Autodesk Inventor part; units mm, degrees
(part 3 of 4)
sketch "스케치34" plane through (0, 0, 0) normal (0, -1, 0) x (1, 0, 0)
  line L0 (50.8787, 118.101) -> (84.8787, 118.101) projected
  arc A0 (87.8787, 115.101) -> (84.8787, 118.101) centre (84.8787, 115.101) ccw projected
  line L1 (87.8787, 115.101) -> (87.8787, 101.101) projected
  arc A1 (84.8787, 98.101) -> (87.8787, 101.101) centre (84.8787, 101.101) ccw projected
  line L2 (84.8787, 98.101) -> (50.8787, 98.101) projected
  arc A2 (47.8787, 101.101) -> (50.8787, 98.101) centre (50.8787, 101.101) ccw projected
  line L3 (47.8787, 101.101) -> (47.8787, 115.101) projected
  arc A3 (50.8787, 118.101) -> (47.8787, 115.101) centre (50.8787, 115.101) ccw projected
  arc A4 (-27.1, -120.9669) -> (-15.1, -132.9669) centre (-15.1, -120.9669) ccw projected
  line L4 (-15.1, -132.9669) -> (115.7787, -132.9669) projected
  arc A5 (115.7787, -132.9669) -> (127.7787, -120.9669) centre (115.7787, -120.9669) ccw projected
  line L5 (127.7787, -120.9669) -> (127.7787, -81.2883) projected
  arc A6 (127.7787, -81.2883) -> (120.2094, -70.1362) centre (115.7787, -81.2883) ccw projected
  line L6 (120.2094, -70.1362) -> (34.6692, -36.1508) projected
  arc A7 (27.1, -24.9988) -> (34.6692, -36.1508) centre (39.1, -24.9988) ccw projected
  line L7 (27.1, 24.9988) -> (27.1, -24.9988) projected
  arc A8 (34.6692, 36.1508) -> (27.1, 24.9988) centre (39.1, 24.9988) ccw projected
  line L8 (34.6692, 36.1508) -> (120.2094, 70.1362) projected
  arc A9 (120.2094, 70.1362) -> (127.7787, 81.2883) centre (115.7787, 81.2883) ccw projected
  line L9 (127.7787, 81.2883) -> (127.7787, 120.9669) projected
  arc A10 (127.7787, 120.9669) -> (115.7787, 132.9669) centre (115.7787, 120.9669) ccw projected
  line L10 (115.7787, 132.9669) -> (-15.1, 132.9669) projected
  arc A11 (-15.1, 132.9669) -> (-27.1, 120.9669) centre (-15.1, 120.9669) ccw projected
  line L11 (-27.1, 120.9669) -> (-27.1, -120.9669) projected
  circle A12 centre (99.9787, -108.101) radius 1.85 projected
  circle A13 centre (15.7787, 108.101) radius 1.85 projected
  circle A14 centre (35.7787, -108.101) radius 1.75 projected
  circle A15 centre (119.9787, 108.101) radius 1.75 projected
  circle A16 centre (119.9787, -108.101) radius 1.75 projected
  circle A17 centre (35.7787, 108.101) radius 1.75 projected
  circle A18 centre (15.7787, -108.101) radius 1.85 projected
  circle A19 centre (99.9787, 108.101) radius 1.85 projected
  circle A20 centre (0, 0) radius 8 projected
  arc A21 (13, 81.501) -> (15, 83.501) centre (13, 83.501) ccw projected
  line L12 (13, 81.501) -> (-13, 81.501) projected
  arc A22 (-15, 83.501) -> (-13, 81.501) centre (-13, 83.501) ccw projected
  line L13 (-15, 83.501) -> (-15, 93.501) projected
  arc A23 (-13, 95.501) -> (-15, 93.501) centre (-13, 93.501) ccw projected
  line L14 (-13, 95.501) -> (13, 95.501) projected
  arc A24 (15, 93.501) -> (13, 95.501) centre (13, 93.501) ccw projected
  line L15 (15, 93.501) -> (15, 83.501) projected
  circle A25 centre (49.8107, 76.501) radius 1.6 projected
  circle A26 centre (39.1, 76.501) radius 1.6 projected
  circle A27 centre (69.8107, 76.501) radius 1.6 projected
  circle A28 centre (89.8107, 76.501) radius 1.6 projected
  circle A29 centre (-4.9749, 12.0104) radius 3.1 projected
  circle A30 centre (4.9749, 12.0104) radius 3.1 projected
  circle A31 centre (-12.0104, 4.9749) radius 3.1 projected
  circle A32 centre (12.0104, 4.9749) radius 3.1 projected
  circle A33 centre (9.1, 76.501) radius 1.6 projected
  circle A34 centre (-10.9, 76.501) radius 1.6 projected
  circle A35 centre (39.1, -76.501) radius 1.6 projected
  circle A36 centre (49.8107, -76.501) radius 1.6 projected
  circle A37 centre (9.1, -76.501) radius 1.6 projected
  circle A38 centre (-10.9, -76.501) radius 1.6 projected
  circle A39 centre (69.8107, -76.501) radius 1.6 projected
  circle A40 centre (89.8107, -76.501) radius 1.6 projected
  circle A41 centre (-12.0104, -4.9749) radius 1.6 projected
  circle A42 centre (4.9749, -12.0104) radius 1.6 projected
  circle A43 centre (12.0104, -4.9749) radius 1.6 projected
  circle A44 centre (-4.9749, -12.0104) radius 1.6 projected
  line L16 (15, -83.501) -> (15, -93.501) projected
  arc A45 (13, -95.501) -> (15, -93.501) centre (13, -93.501) ccw projected
  line L17 (13, -95.501) -> (-13, -95.501) projected
  arc A46 (-15, -93.501) -> (-13, -95.501) centre (-13, -93.501) ccw projected
  line L18 (-15, -93.501) -> (-15, -83.501) projected
  arc A47 (-13, -81.501) -> (-15, -83.501) centre (-13, -83.501) ccw projected
  line L19 (-13, -81.501) -> (13, -81.501) projected
  arc A48 (15, -83.501) -> (13, -81.501) centre (13, -83.501) ccw projected
  circle A49 centre (114.8107, 76.501) radius 1.6
  line L20 (114.8107, 76.501) -> (114.8107, 78.501)
  line L21 (114.8107, 126.501) -> (114.8107, 128.501)
  line L22 (114.8107, 102.501) -> (-27.1, 102.501)
  line L23 (-27.1, 120.9669) -> (-27.1, -120.9669) projected
  circle A50 centre (89.8107, 76.501) radius 1.6 projected
  circle A51 centre (89.8107, 76.501) radius 1.6
  circle A52 centre (69.8107, 76.501) radius 1.6
  circle A53 centre (49.8107, 76.501) radius 1.6 projected
  circle A54 centre (49.8107, 76.501) radius 1.6
  circle A55 centre (39.1, 76.501) radius 1.6 projected
  circle A56 centre (39.1, 76.501) radius 1.6
  circle A57 centre (9.1, 76.501) radius 1.6 projected
  circle A58 centre (9.1, 76.501) radius 1.6
  circle A59 centre (-10.9, 76.501) radius 1.6 projected
  circle A60 centre (-10.9, 76.501) radius 1.6
  circle A61 centre (114.8107, 128.501) radius 1.6
  circle A62 centre (89.8107, 128.501) radius 1.6
  line L24 (114.8107, 128.501) -> (-24.4401, 128.501) construction
  arc A63 (-15.1, 132.9669) -> (-27.1, 120.9669) centre (-15.1, 120.9669) ccw projected
  circle A64 centre (69.8107, 128.501) radius 1.6
  circle A65 centre (49.8107, 128.501) radius 1.6
  circle A66 centre (34.8107, 128.501) radius 1.6
  circle A67 centre (4.8107, 128.501) radius 1.6
  circle A68 centre (-15.1893, 128.501) radius 1.6
  point P0 (114.8107, 127.501)
  dimension "d223" = 16.2
  dimension "d225" = 20
  dimension "d227" = 3.2
  dimension "d228" = 25
  dimension "d233" = 2
  dimension "d235" = 2
  dimension "d236" = 3.2
  dimension "d237" = 3.2
  dimension "d238" = 25
  dimension "d239" = 20
  dimension "d240" = 30
  dimension "d241" = 15
  dimension "d242" = 20
  dimension "d243" = 20
  dimension "d337" = 4.4659
  constraints: 14 centre point, 8 end point, 7 coincident, 7 point on line, 6 equal radius, 1 horizontal, 1 midpoint, 1 perpendicular, 1 point on circle, 1 vertical
  measures "d223" distance from line of L11 A34.centre
  measures "d225" distance of A28.centre A27.centre
  measures "d227" diameter of A49
  measures "d228" distance of A28.centre L20.start
  measures "d233" distance of L20.start L20.end
  measures "d235" distance of L21.start L21.end
  measures "d236" diameter of A61
  measures "d237" diameter of A62
  measures "d238" horizontal distance of point (114.811, 127.501) A62.centre
  measures "d239" distance of A67.centre A68.centre
  measures "d240" distance of A66.centre A67.centre
  measures "d241" distance of A65.centre A66.centre
  measures "d242" distance of A64.centre A65.centre
  measures "d243" distance of A62.centre A64.centre
  measures "d337" distance from line of L10 A68.centre
extrude "돌출38" cut sketch "스케치34" against normal blind 5 contours A49 | A61 | A62 | A64 | A65 | A66 | A67 | A68
mirror "미러1" about plane through (0, 0, 0) normal (0, 0, 1) of "돌출36"
mirror "미러2" about plane through (0, 0, 0) normal (0, 0, 1) of "돌출35"
mirror "미러3" about plane through (0, 0, 0) normal (0, 0, 1) of "돌출38"
fillet "모깎기8" radius 3 4 edges at (87.8787, 1.5, -98.101) (87.8787, 1.5, -118.101) (47.8787, 1.5, -98.101) (47.8787, 1.5, -118.101)
sketch "스케치35" plane through (0, 0, 0) normal (0, -1, 0) x (1, 0, 0)
  circle A0 centre (69.8107, -128.501) radius 1.6 projected
  circle A1 centre (-15.1893, -128.501) radius 1.6 projected
  circle A2 centre (4.8107, -128.501) radius 1.6 projected
  circle A3 centre (89.8107, -128.501) radius 1.6 projected
  circle A4 centre (49.8107, -128.501) radius 1.6 projected
  circle A5 centre (114.8107, -76.501) radius 1.6 projected
  circle A6 centre (34.8107, -128.501) radius 1.6 projected
  circle A7 centre (114.8107, -128.501) radius 1.6 projected
  line L0 (84.8787, -118.101) -> (50.8787, -118.101) projected
  arc A8 (47.8787, -115.101) -> (50.8787, -118.101) centre (50.8787, -115.101) ccw projected
  line L1 (47.8787, -115.101) -> (47.8787, -101.101) projected
  arc A9 (50.8787, -98.101) -> (47.8787, -101.101) centre (50.8787, -101.101) ccw projected
  line L2 (50.8787, -98.101) -> (84.8787, -98.101) projected
  arc A10 (87.8787, -101.101) -> (84.8787, -98.101) centre (84.8787, -101.101) ccw projected
  line L3 (87.8787, -101.101) -> (87.8787, -115.101) projected
  arc A11 (84.8787, -118.101) -> (87.8787, -115.101) centre (84.8787, -115.101) ccw projected
  circle A12 centre (69.8107, 128.501) radius 1.6 projected
  circle A13 centre (-15.1893, 128.501) radius 1.6 projected
  circle A14 centre (4.8107, 128.501) radius 1.6 projected
  circle A15 centre (89.8107, 128.501) radius 1.6 projected
  circle A16 centre (49.8107, 128.501) radius 1.6 projected
  circle A17 centre (114.8107, 76.501) radius 1.6 projected
  circle A18 centre (34.8107, 128.501) radius 1.6 projected
  circle A19 centre (114.8107, 128.501) radius 1.6 projected
  line L4 (50.8787, 118.101) -> (84.8787, 118.101) projected
  arc A20 (87.8787, 115.101) -> (84.8787, 118.101) centre (84.8787, 115.101) ccw projected
  line L5 (87.8787, 115.101) -> (87.8787, 101.101) projected
  arc A21 (84.8787, 98.101) -> (87.8787, 101.101) centre (84.8787, 101.101) ccw projected
  line L6 (84.8787, 98.101) -> (50.8787, 98.101) projected
  arc A22 (47.8787, 101.101) -> (50.8787, 98.101) centre (50.8787, 101.101) ccw projected
  line L7 (47.8787, 101.101) -> (47.8787, 115.101) projected
  arc A23 (50.8787, 118.101) -> (47.8787, 115.101) centre (50.8787, 115.101) ccw projected
  arc A24 (-27.1, -120.9669) -> (-15.1, -132.9669) centre (-15.1, -120.9669) ccw projected
  line L8 (-15.1, -132.9669) -> (115.7787, -132.9669) projected
  arc A25 (115.7787, -132.9669) -> (127.7787, -120.9669) centre (115.7787, -120.9669) ccw projected
  line L9 (127.7787, -120.9669) -> (127.7787, -81.2883) projected
  arc A26 (127.7787, -81.2883) -> (120.2094, -70.1362) centre (115.7787, -81.2883) ccw projected
  line L10 (120.2094, -70.1362) -> (34.6692, -36.1508) projected
  arc A27 (27.1, -24.9988) -> (34.6692, -36.1508) centre (39.1, -24.9988) ccw projected
  line L11 (27.1, 24.9988) -> (27.1, -24.9988) projected
  arc A28 (34.6692, 36.1508) -> (27.1, 24.9988) centre (39.1, 24.9988) ccw projected
  line L12 (34.6692, 36.1508) -> (120.2094, 70.1362) projected
  arc A29 (120.2094, 70.1362) -> (127.7787, 81.2883) centre (115.7787, 81.2883) ccw projected
  line L13 (127.7787, 81.2883) -> (127.7787, 120.9669) projected
  arc A30 (127.7787, 120.9669) -> (115.7787, 132.9669) centre (115.7787, 120.9669) ccw projected
  line L14 (115.7787, 132.9669) -> (-15.1, 132.9669) projected
  arc A31 (-15.1, 132.9669) -> (-27.1, 120.9669) centre (-15.1, 120.9669) ccw projected
  line L15 (-27.1, 120.9669) -> (-27.1, -120.9669) projected
  circle A32 centre (99.9787, -108.101) radius 1.85 projected
  circle A33 centre (15.7787, 108.101) radius 1.85 projected
  circle A34 centre (35.7787, -108.101) radius 1.75 projected
  circle A35 centre (119.9787, 108.101) radius 1.75 projected
  circle A36 centre (119.9787, -108.101) radius 1.75 projected
  circle A37 centre (35.7787, 108.101) radius 1.75 projected
  circle A38 centre (15.7787, -108.101) radius 1.85 projected
  circle A39 centre (99.9787, 108.101) radius 1.85 projected
  circle A40 centre (0, 0) radius 8 projected
  arc A41 (13, 81.501) -> (15, 83.501) centre (13, 83.501) ccw projected
  line L16 (13, 81.501) -> (-13, 81.501) projected
  arc A42 (-15, 83.501) -> (-13, 81.501) centre (-13, 83.501) ccw projected
  line L17 (-15, 83.501) -> (-15, 93.501) projected
  arc A43 (-13, 95.501) -> (-15, 93.501) centre (-13, 93.501) ccw projected
  line L18 (-13, 95.501) -> (13, 95.501) projected
  arc A44 (15, 93.501) -> (13, 95.501) centre (13, 93.501) ccw projected
  line L19 (15, 93.501) -> (15, 83.501) projected
  circle A45 centre (49.8107, 76.501) radius 1.6 projected
  circle A46 centre (39.1, 76.501) radius 1.6 projected
  circle A47 centre (69.8107, 76.501) radius 1.6 projected
  circle A48 centre (89.8107, 76.501) radius 1.6 projected
  circle A49 centre (-4.9749, 12.0104) radius 3.1 projected
  circle A50 centre (4.9749, 12.0104) radius 3.1 projected
  circle A51 centre (-12.0104, 4.9749) radius 3.1 projected
  circle A52 centre (12.0104, 4.9749) radius 3.1 projected
  circle A53 centre (9.1, 76.501) radius 1.6 projected
  circle A54 centre (-10.9, 76.501) radius 1.6 projected
  circle A55 centre (39.1, -76.501) radius 1.6 projected
  circle A56 centre (49.8107, -76.501) radius 1.6 projected
  circle A57 centre (9.1, -76.501) radius 1.6 projected
  circle A58 centre (-10.9, -76.501) radius 1.6 projected
  circle A59 centre (69.8107, -76.501) radius 1.6 projected
  circle A60 centre (89.8107, -76.501) radius 1.6 projected
  circle A61 centre (-12.0104, -4.9749) radius 1.6 projected
  circle A62 centre (4.9749, -12.0104) radius 1.6 projected
  circle A63 centre (12.0104, -4.9749) radius 1.6 projected
  circle A64 centre (-4.9749, -12.0104) radius 1.6 projected
  line L20 (15, -83.501) -> (15, -93.501) projected
  arc A65 (13, -95.501) -> (15, -93.501) centre (13, -93.501) ccw projected
  line L21 (13, -95.501) -> (-13, -95.501) projected
  arc A66 (-15, -93.501) -> (-13, -95.501) centre (-13, -93.501) ccw projected
  line L22 (-15, -93.501) -> (-15, -83.501) projected
  arc A67 (-13, -81.501) -> (-15, -83.501) centre (-13, -83.501) ccw projected
  line L23 (-13, -81.501) -> (13, -81.501) projected
  arc A68 (15, -83.501) -> (13, -81.501) centre (13, -83.501) ccw projected
  circle A69 centre (12.0104, 4.9749) radius 1.6
  circle A70 centre (4.9749, 12.0104) radius 1.6
  circle A71 centre (-4.9749, 12.0104) radius 1.6
  circle A72 centre (-12.0104, 4.9749) radius 3.1 projected
  circle A73 centre (-12.0104, 4.9749) radius 1.6
  dimension "d245" = 3.2
  dimension "d246" = 3.2
  dimension "d247" = 3.2
  dimension "d248" = 3.2
  constraints: 4 centre point, 4 coincident
  measures "d245" diameter of A69
  measures "d246" diameter of A70
  measures "d247" diameter of A71
  measures "d248" diameter of A73
extrude "돌출39" add sketch "스케치35" against normal blind 5 contours A49 | A50 | A51 | A52
sketch "스케치36" plane through (0, 5, 0) normal (0, 1, 0) x (1, 0, 0)
  circle A0 centre (-4.9749, -12.0104) radius 1.6 projected
  circle A1 centre (4.9749, -12.0104) radius 1.6 projected
  circle A2 centre (-12.0104, -4.9749) radius 1.6 projected
  circle A3 centre (12.0104, -4.9749) radius 1.6 projected
  circle A4 centre (69.8107, 128.501) radius 1.6 projected
  circle A5 centre (-15.1893, 128.501) radius 1.6 projected
  circle A6 centre (4.8107, 128.501) radius 1.6 projected
  circle A7 centre (89.8107, 128.501) radius 1.6 projected
  circle A8 centre (49.8107, 128.501) radius 1.6 projected
  circle A9 centre (114.8107, 76.501) radius 1.6 projected
  circle A10 centre (34.8107, 128.501) radius 1.6 projected
  circle A11 centre (114.8107, 128.501) radius 1.6 projected
  circle A12 centre (77.8787, 108.101) radius 1.8 projected
  circle A13 centre (57.8787, 108.101) radius 1.8 projected
  circle A14 centre (69.8107, -128.501) radius 1.6 projected
  circle A15 centre (-15.1893, -128.501) radius 1.6 projected
  circle A16 centre (4.8107, -128.501) radius 1.6 projected
  circle A17 centre (89.8107, -128.501) radius 1.6 projected
  circle A18 centre (49.8107, -128.501) radius 1.6 projected
  circle A19 centre (114.8107, -76.501) radius 1.6 projected
  circle A20 centre (34.8107, -128.501) radius 1.6 projected
  circle A21 centre (114.8107, -128.501) radius 1.6 projected
  circle A22 centre (77.8787, -108.101) radius 1.8 projected
  circle A23 centre (57.8787, -108.101) radius 1.8 projected
  circle A24 centre (99.9787, 108.101) radius 1.85 projected
  circle A25 centre (15.7787, -108.101) radius 1.85 projected
  circle A26 centre (35.7787, 108.101) radius 1.75 projected
  circle A27 centre (119.9787, -108.101) radius 1.75 projected
  circle A28 centre (119.9787, 108.101) radius 1.75 projected
  circle A29 centre (35.7787, -108.101) radius 1.75 projected
  circle A30 centre (15.7787, 108.101) radius 1.85 projected
  circle A31 centre (99.9787, -108.101) radius 1.85 projected
  arc A32 (-15.1, 132.9669) -> (-27.1, 120.9669) centre (-15.1, 120.9669) ccw projected
  line L0 (-27.1, 120.9669) -> (-27.1, -120.9669) projected
  arc A33 (-27.1, -120.9669) -> (-15.1, -132.9669) centre (-15.1, -120.9669) ccw projected
  line L1 (-15.1, -132.9669) -> (115.7787, -132.9669) projected
  arc A34 (115.7787, -132.9669) -> (127.7787, -120.9669) centre (115.7787, -120.9669) ccw projected
  line L2 (127.7787, -120.9669) -> (127.7787, -81.2883) projected
  arc A35 (127.7787, -81.2883) -> (120.2094, -70.1362) centre (115.7787, -81.2883) ccw projected
  line L3 (120.2094, -70.1362) -> (34.6692, -36.1508) projected
  arc A36 (27.1, -24.9988) -> (34.6692, -36.1508) centre (39.1, -24.9988) ccw projected
  line L4 (27.1, -24.9988) -> (27.1, 24.9988) projected
  arc A37 (34.6692, 36.1508) -> (27.1, 24.9988) centre (39.1, 24.9988) ccw projected
  line L5 (34.6692, 36.1508) -> (120.2094, 70.1362) projected
  arc A38 (120.2094, 70.1362) -> (127.7787, 81.2883) centre (115.7787, 81.2883) ccw projected
  line L6 (127.7787, 81.2883) -> (127.7787, 120.9669) projected
  arc A39 (127.7787, 120.9669) -> (115.7787, 132.9669) centre (115.7787, 120.9669) ccw projected
  line L7 (115.7787, 132.9669) -> (-15.1, 132.9669) projected
  arc A40 (15, -83.501) -> (13, -81.501) centre (13, -83.501) ccw projected
  line L8 (15, -83.501) -> (15, -93.501) projected
  arc A41 (13, -95.501) -> (15, -93.501) centre (13, -93.501) ccw projected
  line L9 (13, -95.501) -> (-13, -95.501) projected
  arc A42 (-15, -93.501) -> (-13, -95.501) centre (-13, -93.501) ccw projected
  line L10 (-15, -93.501) -> (-15, -83.501) projected
  arc A43 (-13, -81.501) -> (-15, -83.501) centre (-13, -83.501) ccw projected
  line L11 (-13, -81.501) -> (13, -81.501) projected
  circle A44 centre (49.8107, -76.501) radius 1.6 projected
  circle A45 centre (39.1, -76.501) radius 1.6 projected
  circle A46 centre (69.8107, -76.501) radius 1.6 projected
  circle A47 centre (89.8107, -76.501) radius 1.6 projected
  circle A48 centre (9.1, -76.501) radius 1.6 projected
  circle A49 centre (-10.9, -76.501) radius 1.6 projected
  circle A50 centre (0, 0) radius 8 projected
  line L12 (15, 93.501) -> (15, 83.501) projected
  arc A51 (13, 81.501) -> (15, 83.501) centre (13, 83.501) ccw projected
  line L13 (13, 81.501) -> (-13, 81.501) projected
  arc A52 (-15, 83.501) -> (-13, 81.501) centre (-13, 83.501) ccw projected
  line L14 (-15, 83.501) -> (-15, 93.501) projected
  arc A53 (-13, 95.501) -> (-15, 93.501) centre (-13, 93.501) ccw projected
  line L15 (-13, 95.501) -> (13, 95.501) projected
  arc A54 (15, 93.501) -> (13, 95.501) centre (13, 93.501) ccw projected
  circle A55 centre (39.1, 76.501) radius 1.6 projected
  circle A56 centre (49.8107, 76.501) radius 1.6 projected
  circle A57 centre (9.1, 76.501) radius 1.6 projected
  circle A58 centre (-10.9, 76.501) radius 1.6 projected
  circle A59 centre (69.8107, 76.501) radius 1.6 projected
  circle A60 centre (89.8107, 76.501) radius 1.6 projected
  circle A61 centre (12.0104, 4.9749) radius 3.1 projected
  circle A62 centre (-4.9749, 12.0104) radius 3.1 projected
  circle A63 centre (-12.0104, 4.9749) radius 3.1 projected
  circle A64 centre (4.9749, 12.0104) radius 3.1 projected
extrude "돌출40" add sketch "스케치36" against normal blind 5 contours A19 | A44 | A45 | A46 | A47 | A48 | A49
sketch "스케치39" plane through (0, 5, 0) normal (0, 1, 0) x (1, 0, 0)
  circle A0 centre (-4.9749, -12.0104) radius 1.6 projected
  circle A1 centre (4.9749, -12.0104) radius 1.6 projected
  circle A2 centre (-12.0104, -4.9749) radius 1.6 projected
  circle A3 centre (12.0104, -4.9749) radius 1.6 projected
  circle A4 centre (69.8107, 128.501) radius 1.6 projected
  circle A5 centre (-15.1893, 128.501) radius 1.6 projected
  circle A6 centre (4.8107, 128.501) radius 1.6 projected
  circle A7 centre (89.8107, 128.501) radius 1.6 projected
  circle A8 centre (49.8107, 128.501) radius 1.6 projected
  circle A9 centre (114.8107, 76.501) radius 1.6 projected
  circle A10 centre (34.8107, 128.501) radius 1.6 projected
  circle A11 centre (114.8107, 128.501) radius 1.6 projected
  circle A12 centre (77.8787, 108.101) radius 1.8 projected
  circle A13 centre (57.8787, 108.101) radius 1.8 projected
  circle A14 centre (69.8107, -128.501) radius 1.6 projected
  circle A15 centre (-15.1893, -128.501) radius 1.6 projected
  circle A16 centre (4.8107, -128.501) radius 1.6 projected
  circle A17 centre (89.8107, -128.501) radius 1.6 projected
  circle A18 centre (49.8107, -128.501) radius 1.6 projected
  circle A19 centre (34.8107, -128.501) radius 1.6 projected
  circle A20 centre (114.8107, -128.501) radius 1.6 projected
  circle A21 centre (77.8787, -108.101) radius 1.8 projected
  circle A22 centre (57.8787, -108.101) radius 1.8 projected
  circle A23 centre (99.9787, 108.101) radius 1.85 projected
  circle A24 centre (15.7787, -108.101) radius 1.85 projected
  circle A25 centre (35.7787, 108.101) radius 1.75 projected
  circle A26 centre (119.9787, -108.101) radius 1.75 projected
  circle A27 centre (119.9787, 108.101) radius 1.75 projected
  circle A28 centre (35.7787, -108.101) radius 1.75 projected
  circle A29 centre (15.7787, 108.101) radius 1.85 projected
  circle A30 centre (99.9787, -108.101) radius 1.85 projected
  arc A31 (-15.1, 132.9669) -> (-27.1, 120.9669) centre (-15.1, 120.9669) ccw projected
  line L0 (-27.1, 120.9669) -> (-27.1, -120.9669) projected
  arc A32 (-27.1, -120.9669) -> (-15.1, -132.9669) centre (-15.1, -120.9669) ccw projected
  line L1 (-15.1, -132.9669) -> (115.7787, -132.9669) projected
  arc A33 (115.7787, -132.9669) -> (127.7787, -120.9669) centre (115.7787, -120.9669) ccw projected
  line L2 (127.7787, -120.9669) -> (127.7787, -81.2883) projected
  arc A34 (127.7787, -81.2883) -> (120.2094, -70.1362) centre (115.7787, -81.2883) ccw projected
  line L3 (120.2094, -70.1362) -> (34.6692, -36.1508) projected
  arc A35 (27.1, -24.9988) -> (34.6692, -36.1508) centre (39.1, -24.9988) ccw projected
  line L4 (27.1, -24.9988) -> (27.1, 24.9988) projected
  arc A36 (34.6692, 36.1508) -> (27.1, 24.9988) centre (39.1, 24.9988) ccw projected
  line L5 (34.6692, 36.1508) -> (120.2094, 70.1362) projected
  arc A37 (120.2094, 70.1362) -> (127.7787, 81.2883) centre (115.7787, 81.2883) ccw projected
  line L6 (127.7787, 81.2883) -> (127.7787, 120.9669) projected
  arc A38 (127.7787, 120.9669) -> (115.7787, 132.9669) centre (115.7787, 120.9669) ccw projected
  line L7 (115.7787, 132.9669) -> (-15.1, 132.9669) projected
  arc A39 (15, -83.501) -> (13, -81.501) centre (13, -83.501) ccw projected
  line L8 (15, -83.501) -> (15, -93.501) projected
  arc A40 (13, -95.501) -> (15, -93.501) centre (13, -93.501) ccw projected
  line L9 (13, -95.501) -> (-13, -95.501) projected
  arc A41 (-15, -93.501) -> (-13, -95.501) centre (-13, -93.501) ccw projected
  line L10 (-15, -93.501) -> (-15, -83.501) projected
  arc A42 (-13, -81.501) -> (-15, -83.501) centre (-13, -83.501) ccw projected
  line L11 (-13, -81.501) -> (13, -81.501) projected
  circle A43 centre (0, 0) radius 8 projected
  line L12 (15, 93.501) -> (15, 83.501) projected
  arc A44 (13, 81.501) -> (15, 83.501) centre (13, 83.501) ccw projected
  line L13 (13, 81.501) -> (-13, 81.501) projected
  arc A45 (-15, 83.501) -> (-13, 81.501) centre (-13, 83.501) ccw projected
  line L14 (-15, 83.501) -> (-15, 93.501) projected
  arc A46 (-13, 95.501) -> (-15, 93.501) centre (-13, 93.501) ccw projected
  line L15 (-13, 95.501) -> (13, 95.501) projected
  arc A47 (15, 93.501) -> (13, 95.501) centre (13, 93.501) ccw projected
  circle A48 centre (39.1, 76.501) radius 1.6 projected
  circle A49 centre (49.8107, 76.501) radius 1.6 projected
  circle A50 centre (9.1, 76.501) radius 1.6 projected
  circle A51 centre (-10.9, 76.501) radius 1.6 projected
  circle A52 centre (69.8107, 76.501) radius 1.6 projected
  circle A53 centre (89.8107, 76.501) radius 1.6 projected
  circle A54 centre (12.0104, 4.9749) radius 3.1 projected
  circle A55 centre (-4.9749, 12.0104) radius 3.1 projected
  circle A56 centre (-12.0104, 4.9749) radius 3.1 projected
  circle A57 centre (4.9749, 12.0104) radius 3.1 projected
  line L16 (-15.1893, -128.501) -> (-15.1893, -126.501)
  line L17 (-15.1893, -126.501) -> (-15.1893, -78.501)
  line L18 (-15.1893, -78.501) -> (-15.1893, -76.501)
  circle A58 centre (-15.1893, -76.501) radius 1.6
  line L19 (-15.1893, -76.501) -> (115.7787, -76.501) construction
  circle A59 centre (4.8107, -76.501) radius 1.6
  circle A60 centre (34.8107, -76.501) radius 1.6
  circle A61 centre (49.8107, -76.501) radius 1.6
  circle A62 centre (69.8107, -76.501) radius 1.6
  circle A63 centre (89.8107, -76.501) radius 1.6
  circle A64 centre (114.8107, -76.501) radius 1.6
  dimension "d292" = 2
  dimension "d293" = 48
  dimension "d294" = 2
  dimension "d295" = 3.2
  constraints: 8 end point, 8 point on line, 7 centre point, 6 equal radius, 6 vertical alignment, 1 coincident, 1 horizontal, 1 vertical
  measures "d292" distance of L16.start L16.end
  measures "d293" distance of L16.end L17.end
  measures "d294" distance of L17.end L18.end
  measures "d295" diameter of A58
extrude "돌출41" cut sketch "스케치39" against normal blind 5 contours A58 | A59 | A60 | A61 | A62 | A63 | A64
sketch "스케치40" plane through (0, 5, 0) normal (0, 1, 0) x (1, 0, 0)
  circle A0 centre (34.8107, -76.501) radius 1.6 projected
  circle A1 centre (114.8107, -76.501) radius 1.6 projected
  circle A2 centre (49.8107, -76.501) radius 1.6 projected
  circle A3 centre (4.8107, -76.501) radius 1.6 projected
  circle A4 centre (89.8107, -76.501) radius 1.6 projected
  circle A5 centre (69.8107, -76.501) radius 1.6 projected
  circle A6 centre (-15.1893, -76.501) radius 1.6 projected
  circle A7 centre (-4.9749, -12.0104) radius 1.6 projected
  circle A8 centre (4.9749, -12.0104) radius 1.6 projected
  circle A9 centre (-12.0104, -4.9749) radius 1.6 projected
  circle A10 centre (12.0104, -4.9749) radius 1.6 projected
  circle A11 centre (69.8107, 128.501) radius 1.6 projected
  circle A12 centre (-15.1893, 128.501) radius 1.6 projected
  circle A13 centre (4.8107, 128.501) radius 1.6 projected
  circle A14 centre (89.8107, 128.501) radius 1.6 projected
  circle A15 centre (49.8107, 128.501) radius 1.6 projected
  circle A16 centre (114.8107, 76.501) radius 1.6 projected
  circle A17 centre (34.8107, 128.501) radius 1.6 projected
  circle A18 centre (114.8107, 128.501) radius 1.6 projected
  circle A19 centre (77.8787, 108.101) radius 1.8 projected
  circle A20 centre (57.8787, 108.101) radius 1.8 projected
  circle A21 centre (69.8107, -128.501) radius 1.6 projected
  circle A22 centre (-15.1893, -128.501) radius 1.6 projected
  circle A23 centre (4.8107, -128.501) radius 1.6 projected
  circle A24 centre (89.8107, -128.501) radius 1.6 projected
  circle A25 centre (49.8107, -128.501) radius 1.6 projected
  circle A26 centre (34.8107, -128.501) radius 1.6 projected
  circle A27 centre (114.8107, -128.501) radius 1.6 projected
  circle A28 centre (77.8787, -108.101) radius 1.8 projected
  circle A29 centre (57.8787, -108.101) radius 1.8 projected
  circle A30 centre (99.9787, 108.101) radius 1.85 projected
  circle A31 centre (15.7787, -108.101) radius 1.85 projected
  circle A32 centre (35.7787, 108.101) radius 1.75 projected
  circle A33 centre (119.9787, -108.101) radius 1.75 projected
  circle A34 centre (119.9787, 108.101) radius 1.75 projected
  circle A35 centre (35.7787, -108.101) radius 1.75 projected
  circle A36 centre (15.7787, 108.101) radius 1.85 projected
  circle A37 centre (99.9787, -108.101) radius 1.85 projected
  arc A38 (-15.1, 132.9669) -> (-27.1, 120.9669) centre (-15.1, 120.9669) ccw projected
  line L0 (-27.1, 120.9669) -> (-27.1, -120.9669) projected
  arc A39 (-27.1, -120.9669) -> (-15.1, -132.9669) centre (-15.1, -120.9669) ccw projected
  line L1 (-15.1, -132.9669) -> (115.7787, -132.9669) projected
  arc A40 (115.7787, -132.9669) -> (127.7787, -120.9669) centre (115.7787, -120.9669) ccw projected
  line L2 (127.7787, -120.9669) -> (127.7787, -81.2883) projected
  arc A41 (127.7787, -81.2883) -> (120.2094, -70.1362) centre (115.7787, -81.2883) ccw projected
  line L3 (120.2094, -70.1362) -> (34.6692, -36.1508) projected
  arc A42 (27.1, -24.9988) -> (34.6692, -36.1508) centre (39.1, -24.9988) ccw projected
  line L4 (27.1, -24.9988) -> (27.1, 24.9988) projected
  arc A43 (34.6692, 36.1508) -> (27.1, 24.9988) centre (39.1, 24.9988) ccw projected
  line L5 (34.6692, 36.1508) -> (120.2094, 70.1362) projected
  arc A44 (120.2094, 70.1362) -> (127.7787, 81.2883) centre (115.7787, 81.2883) ccw projected
  line L6 (127.7787, 81.2883) -> (127.7787, 120.9669) projected
  arc A45 (127.7787, 120.9669) -> (115.7787, 132.9669) centre (115.7787, 120.9669) ccw projected
  line L7 (115.7787, 132.9669) -> (-15.1, 132.9669) projected
  arc A46 (15, -83.501) -> (13, -81.501) centre (13, -83.501) ccw projected
  line L8 (15, -83.501) -> (15, -93.501) projected
  arc A47 (13, -95.501) -> (15, -93.501) centre (13, -93.501) ccw projected
  line L9 (13, -95.501) -> (-13, -95.501) projected
  arc A48 (-15, -93.501) -> (-13, -95.501) centre (-13, -93.501) ccw projected
  line L10 (-15, -93.501) -> (-15, -83.501) projected
  arc A49 (-13, -81.501) -> (-15, -83.501) centre (-13, -83.501) ccw projected
  line L11 (-13, -81.501) -> (13, -81.501) projected
  circle A50 centre (0, 0) radius 8 projected
  line L12 (15, 93.501) -> (15, 83.501) projected
  arc A51 (13, 81.501) -> (15, 83.501) centre (13, 83.501) ccw projected
  line L13 (13, 81.501) -> (-13, 81.501) projected
  arc A52 (-15, 83.501) -> (-13, 81.501) centre (-13, 83.501) ccw projected
  line L14 (-15, 83.501) -> (-15, 93.501) projected
  arc A53 (-13, 95.501) -> (-15, 93.501) centre (-13, 93.501) ccw projected
  line L15 (-13, 95.501) -> (13, 95.501) projected
  arc A54 (15, 93.501) -> (13, 95.501) centre (13, 93.501) ccw projected
  circle A55 centre (39.1, 76.501) radius 1.6 projected
  circle A56 centre (49.8107, 76.501) radius 1.6 projected
  circle A57 centre (9.1, 76.501) radius 1.6 projected
  circle A58 centre (-10.9, 76.501) radius 1.6 projected
  circle A59 centre (69.8107, 76.501) radius 1.6 projected
  circle A60 centre (89.8107, 76.501) radius 1.6 projected
  circle A61 centre (12.0104, 4.9749) radius 3.1 projected
  circle A62 centre (-4.9749, 12.0104) radius 3.1 projected
  circle A63 centre (-12.0104, 4.9749) radius 3.1 projected
  circle A64 centre (4.9749, 12.0104) radius 3.1 projected
extrude "돌출42" add sketch "스케치40" against normal blind 5 contours A11 | A12 | A13 | A14 | A15 | A16 | A17 | A18 | A55 | A56 | A57 | A58 | A59 | A60
mirror "미러4" about plane through (0, 0, 0) normal (0, 0, 1) of "돌출41", "돌출38"
chamfer "모따기4" distance 1.5 angle 45 4 edges at (-13.6104, 5, 4.9749) (-6.5749, 5, 12.0104) (3.3749, 5, 12.0104) (10.4104, 5, 4.9749)
sketch "스케치41" plane through (27.1, 0, 24.9988) normal (1, 0, 0) x (0, 0, -1)
  line L0 (49.9975, 5) -> (49.9975, 0) projected
  line L1 (49.9975, 2.5) -> (-11.1521, 2.5)
  line L2 (-11.1521, 5) -> (-11.1521, 0) projected
  line L3 (0, 0) -> (0, 5) projected
  line L4 (0, 0) -> (49.9975, 0) projected
  line L5 (49.9975, 5) -> (49.9975, 0) projected
  line L6 (0, 5) -> (49.9975, 5) projected
  circle A0 centre (32.9988, 2.5) radius 1.25 projected
  circle A1 centre (42.9988, 2.5) radius 1.25 projected
  circle A2 centre (17, 2.5) radius 1.25
  circle A3 centre (7, 2.5) radius 1.25
  circle A4 centre (32.9988, 2.5) radius 1.25 projected
  point P0 (24.9988, 0)
  point P1 (0, 2.5)
  dimension "d303" = 10
  dimension "d304" = 7
  constraints: 3 midpoint, 2 centre point, 2 end point, 2 equal radius, 2 point on line
  measures "d303" distance of A3.centre A2.centre
  measures "d304" distance of point (0, 2.5) A3.centre
extrude "돌출43" cut sketch "스케치41" against normal blind 6 contours A3 L1 | L1 A3 | A2 L1 | L1 A2
sketch "스케치42" plane through (-27.1, 5, -120.9669) normal (-1, 0, 0) x (0, 0, 1)
  line L0 (0, -5) -> (0, 0) projected
  line L1 (241.9338, -5) -> (0, -5) projected
  line L2 (241.9338, 0) -> (241.9338, -5) projected
  line L3 (0, 0) -> (241.9338, 0) projected
  circle A0 centre (112.9669, -2.5) radius 1.25 projected
  circle A1 centre (102.9669, -2.5) radius 1.25 projected
  circle A2 centre (128.9669, -2.5) radius 1.25
  circle A3 centre (138.9669, -2.5) radius 1.25
  circle A4 centre (112.9669, -2.5) radius 1.25 projected
  point P0 (120.9669, -5)
  dimension "d307" = 10
  dimension "d308" = 16
  constraints: 2 centre point, 2 equal radius
  measures "d307" distance of A3.centre A2.centre
  measures "d308" distance of A0.centre A2.centre
extrude "돌출44" cut sketch "스케치42" against normal blind 6 contours A2 | A3
sketch "스케치44" plane through (0, 0, 0) normal (0, -1, 0) x (1, 0, 0)
  circle A0 centre (114.8107, -128.501) radius 1.6 projected
  circle A1 centre (34.8107, -128.501) radius 1.6 projected
  circle A2 centre (49.8107, -128.501) radius 1.6 projected
  circle A3 centre (89.8107, -128.501) radius 1.6 projected
  circle A4 centre (4.8107, -128.501) radius 1.6 projected
  circle A5 centre (-15.1893, -128.501) radius 1.6 projected
  circle A6 centre (69.8107, -128.501) radius 1.6 projected
  circle A7 centre (-15.1893, -76.501) radius 1.6 projected
  circle A8 centre (69.8107, -76.501) radius 1.6 projected
  circle A9 centre (89.8107, -76.501) radius 1.6 projected
  circle A10 centre (4.8107, -76.501) radius 1.6 projected
  circle A11 centre (49.8107, -76.501) radius 1.6 projected
  circle A12 centre (114.8107, -76.501) radius 1.6 projected
  circle A13 centre (34.8107, -76.501) radius 1.6 projected
  circle A14 centre (34.8107, 76.501) radius 1.6 projected
  circle A15 centre (114.8107, 76.501) radius 1.6 projected
  circle A16 centre (49.8107, 76.501) radius 1.6 projected
  circle A17 centre (4.8107, 76.501) radius 1.6 projected
  circle A18 centre (89.8107, 76.501) radius 1.6 projected
  circle A19 centre (69.8107, 76.501) radius 1.6 projected
  circle A20 centre (-15.1893, 76.501) radius 1.6 projected
  circle A21 centre (-4.9749, 12.0104) radius 1.6 projected
  circle A22 centre (4.9749, 12.0104) radius 1.6 projected
  circle A23 centre (-12.0104, 4.9749) radius 1.6 projected
  circle A24 centre (12.0104, 4.9749) radius 1.6 projected
  line L0 (84.8787, -118.101) -> (50.8787, -118.101) projected
  arc A25 (47.8787, -115.101) -> (50.8787, -118.101) centre (50.8787, -115.101) ccw projected
  line L1 (47.8787, -115.101) -> (47.8787, -101.101) projected
  arc A26 (50.8787, -98.101) -> (47.8787, -101.101) centre (50.8787, -101.101) ccw projected
  line L2 (50.8787, -98.101) -> (84.8787, -98.101) projected
  arc A27 (87.8787, -101.101) -> (84.8787, -98.101) centre (84.8787, -101.101) ccw projected
  line L3 (87.8787, -101.101) -> (87.8787, -115.101) projected
  arc A28 (84.8787, -118.101) -> (87.8787, -115.101) centre (84.8787, -115.101) ccw projected
  circle A29 centre (69.8107, 128.501) radius 1.6 projected
  circle A30 centre (-15.1893, 128.501) radius 1.6 projected
  circle A31 centre (4.8107, 128.501) radius 1.6 projected
  circle A32 centre (89.8107, 128.501) radius 1.6 projected
  circle A33 centre (49.8107, 128.501) radius 1.6 projected
  circle A34 centre (34.8107, 128.501) radius 1.6 projected
  circle A35 centre (114.8107, 128.501) radius 1.6 projected
  line L4 (50.8787, 118.101) -> (84.8787, 118.101) projected
  arc A36 (87.8787, 115.101) -> (84.8787, 118.101) centre (84.8787, 115.101) ccw projected
  line L5 (87.8787, 115.101) -> (87.8787, 101.101) projected
  arc A37 (84.8787, 98.101) -> (87.8787, 101.101) centre (84.8787, 101.101) ccw projected
  line L6 (84.8787, 98.101) -> (50.8787, 98.101) projected
  arc A38 (47.8787, 101.101) -> (50.8787, 98.101) centre (50.8787, 101.101) ccw projected
  line L7 (47.8787, 101.101) -> (47.8787, 115.101) projected
  arc A39 (50.8787, 118.101) -> (47.8787, 115.101) centre (50.8787, 115.101) ccw projected
  arc A40 (-27.1, -120.9669) -> (-15.1, -132.9669) centre (-15.1, -120.9669) ccw projected
  line L8 (-15.1, -132.9669) -> (115.7787, -132.9669) projected
  arc A41 (115.7787, -132.9669) -> (127.7787, -120.9669) centre (115.7787, -120.9669) ccw projected
  line L9 (127.7787, -120.9669) -> (127.7787, -81.2883) projected
  arc A42 (127.7787, -81.2883) -> (120.2094, -70.1362) centre (115.7787, -81.2883) ccw projected
  line L10 (120.2094, -70.1362) -> (34.6692, -36.1508) projected
  arc A43 (27.1, -24.9988) -> (34.6692, -36.1508) centre (39.1, -24.9988) ccw projected
  line L11 (27.1, 24.9988) -> (27.1, -24.9988) projected
  arc A44 (34.6692, 36.1508) -> (27.1, 24.9988) centre (39.1, 24.9988) ccw projected
  line L12 (34.6692, 36.1508) -> (120.2094, 70.1362) projected
  arc A45 (120.2094, 70.1362) -> (127.7787, 81.2883) centre (115.7787, 81.2883) ccw projected
  line L13 (127.7787, 81.2883) -> (127.7787, 120.9669) projected
  arc A46 (127.7787, 120.9669) -> (115.7787, 132.9669) centre (115.7787, 120.9669) ccw projected
  line L14 (115.7787, 132.9669) -> (-15.1, 132.9669) projected
  arc A47 (-15.1, 132.9669) -> (-27.1, 120.9669) centre (-15.1, 120.9669) ccw projected
  line L15 (-27.1, 120.9669) -> (-27.1, -120.9669) projected
  circle A48 centre (99.9787, -108.101) radius 1.85 projected
  circle A49 centre (15.7787, 108.101) radius 1.85 projected
  circle A50 centre (35.7787, -108.101) radius 1.75 projected
  circle A51 centre (119.9787, 108.101) radius 1.75 projected
  circle A52 centre (119.9787, -108.101) radius 1.75 projected
  circle A53 centre (35.7787, 108.101) radius 1.75 projected
  circle A54 centre (15.7787, -108.101) radius 1.85 projected
  circle A55 centre (99.9787, 108.101) radius 1.85 projected
  circle A56 centre (0, 0) radius 8 projected
  arc A57 (13, 81.501) -> (15, 83.501) centre (13, 83.501) ccw projected
  line L16 (13, 81.501) -> (-13, 81.501) projected
  arc A58 (-15, 83.501) -> (-13, 81.501) centre (-13, 83.501) ccw projected
  line L17 (-15, 83.501) -> (-15, 93.501) projected
  arc A59 (-13, 95.501) -> (-15, 93.501) centre (-13, 93.501) ccw projected
  line L18 (-13, 95.501) -> (13, 95.501) projected
  arc A60 (15, 93.501) -> (13, 95.501) centre (13, 93.501) ccw projected
  line L19 (15, 93.501) -> (15, 83.501) projected
  circle A61 centre (-12.0104, -4.9749) radius 1.6 projected
  circle A62 centre (4.9749, -12.0104) radius 1.6 projected
  circle A63 centre (12.0104, -4.9749) radius 1.6 projected
  circle A64 centre (-4.9749, -12.0104) radius 1.6 projected
  line L20 (15, -83.501) -> (15, -93.501) projected
  arc A65 (13, -95.501) -> (15, -93.501) centre (13, -93.501) ccw projected
  line L21 (13, -95.501) -> (-13, -95.501) projected
  arc A66 (-15, -93.501) -> (-13, -95.501) centre (-13, -93.501) ccw projected
  line L22 (-15, -93.501) -> (-15, -83.501) projected
  arc A67 (-13, -81.501) -> (-15, -83.501) centre (-13, -83.501) ccw projected
  line L23 (-13, -81.501) -> (13, -81.501) projected
  arc A68 (15, -83.501) -> (13, -81.501) centre (13, -83.501) ccw projected
  circle A69 centre (-15.1893, 76.501) radius 1.6 projected
  line L24 (-15.1893, 76.501) -> (-15.1893, 74.501)
  circle A70 centre (-18.1, 59.001) radius 1.6
  circle A71 centre (17.9, 59.001) radius 1.6
  dimension "d311" = 2
  dimension "d314" = 3.2
  dimension "d315" = 3.2
  dimension "d320" = 9
  dimension "d321" = 36
  dimension "d322" = 17.5
  constraints: 2 centre point, 2 end point, 1 vertical
  measures "d311" distance of L24.start L24.end
  measures "d314" diameter of A70
  measures "d315" diameter of A71
  measures "d320" distance from line of L15 A70.centre
  measures "d321" distance of A71.centre A70.centre
  measures "d322" vertical distance of A20.centre A70.centre
extrude "돌출45" cut sketch "스케치44" against normal blind 6 contours A70 | A71
sketch "스케치45" plane through (0, 0, 0) normal (0, -1, 0) x (1, 0, 0)
  circle A0 centre (-18.1, 59.001) radius 1.6 projected
  circle A1 centre (17.9, 59.001) radius 1.6 projected
  circle A2 centre (114.8107, -128.501) radius 1.6 projected
  circle A3 centre (34.8107, -128.501) radius 1.6 projected
  circle A4 centre (49.8107, -128.501) radius 1.6 projected
  circle A5 centre (89.8107, -128.501) radius 1.6 projected
  circle A6 centre (4.8107, -128.501) radius 1.6 projected
  circle A7 centre (-15.1893, -128.501) radius 1.6 projected
  circle A8 centre (69.8107, -128.501) radius 1.6 projected
  circle A9 centre (-15.1893, -76.501) radius 1.6 projected
  circle A10 centre (69.8107, -76.501) radius 1.6 projected
  circle A11 centre (89.8107, -76.501) radius 1.6 projected
  circle A12 centre (4.8107, -76.501) radius 1.6 projected
  circle A13 centre (49.8107, -76.501) radius 1.6 projected
  circle A14 centre (114.8107, -76.501) radius 1.6 projected
  circle A15 centre (34.8107, -76.501) radius 1.6 projected
  circle A16 centre (34.8107, 76.501) radius 1.6 projected
  circle A17 centre (114.8107, 76.501) radius 1.6 projected
  circle A18 centre (49.8107, 76.501) radius 1.6 projected
  circle A19 centre (4.8107, 76.501) radius 1.6 projected
  circle A20 centre (89.8107, 76.501) radius 1.6 projected
  circle A21 centre (69.8107, 76.501) radius 1.6 projected
  circle A22 centre (-15.1893, 76.501) radius 1.6 projected
  circle A23 centre (-4.9749, 12.0104) radius 1.6 projected
  circle A24 centre (4.9749, 12.0104) radius 1.6 projected
  circle A25 centre (-12.0104, 4.9749) radius 1.6 projected
  circle A26 centre (12.0104, 4.9749) radius 1.6 projected
  line L0 (84.8787, -118.101) -> (50.8787, -118.101) projected
  arc A27 (47.8787, -115.101) -> (50.8787, -118.101) centre (50.8787, -115.101) ccw projected
  line L1 (47.8787, -115.101) -> (47.8787, -101.101) projected
  arc A28 (50.8787, -98.101) -> (47.8787, -101.101) centre (50.8787, -101.101) ccw projected
  line L2 (50.8787, -98.101) -> (84.8787, -98.101) projected
  arc A29 (87.8787, -101.101) -> (84.8787, -98.101) centre (84.8787, -101.101) ccw projected
  line L3 (87.8787, -101.101) -> (87.8787, -115.101) projected
  arc A30 (84.8787, -118.101) -> (87.8787, -115.101) centre (84.8787, -115.101) ccw projected
  circle A31 centre (69.8107, 128.501) radius 1.6 projected
  circle A32 centre (-15.1893, 128.501) radius 1.6 projected
  circle A33 centre (4.8107, 128.501) radius 1.6 projected
  circle A34 centre (89.8107, 128.501) radius 1.6 projected
  circle A35 centre (49.8107, 128.501) radius 1.6 projected
  circle A36 centre (34.8107, 128.501) radius 1.6 projected
  circle A37 centre (114.8107, 128.501) radius 1.6 projected
  line L4 (50.8787, 118.101) -> (84.8787, 118.101) projected
  arc A38 (87.8787, 115.101) -> (84.8787, 118.101) centre (84.8787, 115.101) ccw projected
  line L5 (87.8787, 115.101) -> (87.8787, 101.101) projected
  arc A39 (84.8787, 98.101) -> (87.8787, 101.101) centre (84.8787, 101.101) ccw projected
  line L6 (84.8787, 98.101) -> (50.8787, 98.101) projected
  arc A40 (47.8787, 101.101) -> (50.8787, 98.101) centre (50.8787, 101.101) ccw projected
  line L7 (47.8787, 101.101) -> (47.8787, 115.101) projected
  arc A41 (50.8787, 118.101) -> (47.8787, 115.101) centre (50.8787, 115.101) ccw projected
  arc A42 (-27.1, -120.9669) -> (-15.1, -132.9669) centre (-15.1, -120.9669) ccw projected
  line L8 (-15.1, -132.9669) -> (115.7787, -132.9669) projected
  arc A43 (115.7787, -132.9669) -> (127.7787, -120.9669) centre (115.7787, -120.9669) ccw projected
  line L9 (127.7787, -120.9669) -> (127.7787, -81.2883) projected
  arc A44 (127.7787, -81.2883) -> (120.2094, -70.1362) centre (115.7787, -81.2883) ccw projected
  line L10 (120.2094, -70.1362) -> (34.6692, -36.1508) projected
  arc A45 (27.1, -24.9988) -> (34.6692, -36.1508) centre (39.1, -24.9988) ccw projected
  line L11 (27.1, 24.9988) -> (27.1, -24.9988) projected
  arc A46 (34.6692, 36.1508) -> (27.1, 24.9988) centre (39.1, 24.9988) ccw projected
  line L12 (34.6692, 36.1508) -> (120.2094, 70.1362) projected
  arc A47 (120.2094, 70.1362) -> (127.7787, 81.2883) centre (115.7787, 81.2883) ccw projected
  line L13 (127.7787, 81.2883) -> (127.7787, 120.9669) projected
  arc A48 (127.7787, 120.9669) -> (115.7787, 132.9669) centre (115.7787, 120.9669) ccw projected
  line L14 (115.7787, 132.9669) -> (-15.1, 132.9669) projected
  arc A49 (-15.1, 132.9669) -> (-27.1, 120.9669) centre (-15.1, 120.9669) ccw projected
  line L15 (-27.1, 120.9669) -> (-27.1, -120.9669) projected
  circle A50 centre (99.9787, -108.101) radius 1.85 projected
  circle A51 centre (15.7787, 108.101) radius 1.85 projected
  circle A52 centre (35.7787, -108.101) radius 1.75 projected
  circle A53 centre (119.9787, 108.101) radius 1.75 projected
  circle A54 centre (119.9787, -108.101) radius 1.75 projected
  circle A55 centre (35.7787, 108.101) radius 1.75 projected
  circle A56 centre (15.7787, -108.101) radius 1.85 projected
  circle A57 centre (99.9787, 108.101) radius 1.85 projected
  circle A58 centre (0, 0) radius 8 projected
  arc A59 (13, 81.501) -> (15, 83.501) centre (13, 83.501) ccw projected
  line L16 (13, 81.501) -> (-13, 81.501) projected
  arc A60 (-15, 83.501) -> (-13, 81.501) centre (-13, 83.501) ccw projected
  line L17 (-15, 83.501) -> (-15, 93.501) projected
  arc A61 (-13, 95.501) -> (-15, 93.501) centre (-13, 93.501) ccw projected
  line L18 (-13, 95.501) -> (13, 95.501) projected
  arc A62 (15, 93.501) -> (13, 95.501) centre (13, 93.501) ccw projected
  line L19 (15, 93.501) -> (15, 83.501) projected
  circle A63 centre (-12.0104, -4.9749) radius 1.6 projected
  circle A64 centre (4.9749, -12.0104) radius 1.6 projected
  circle A65 centre (12.0104, -4.9749) radius 1.6 projected
  circle A66 centre (-4.9749, -12.0104) radius 1.6 projected
  line L20 (15, -83.501) -> (15, -93.501) projected
  arc A67 (13, -95.501) -> (15, -93.501) centre (13, -93.501) ccw projected
  line L21 (13, -95.501) -> (-13, -95.501) projected
  arc A68 (-15, -93.501) -> (-13, -95.501) centre (-13, -93.501) ccw projected
  line L22 (-15, -93.501) -> (-15, -83.501) projected
  arc A69 (-13, -81.501) -> (-15, -83.501) centre (-13, -83.501) ccw projected
  line L23 (-13, -81.501) -> (13, -81.501) projected
  arc A70 (15, -83.501) -> (13, -81.501) centre (13, -83.501) ccw projected
  line L24 (-27.1, 0) -> (-27.1, -28.2)
  line L25 (-27.1, -120.9669) -> (-27.1, 120.9669) projected
  line L26 (-27.1, 0) -> (-27.1, 28.2)
  arc A71 (127.7787, 120.9669) -> (115.7787, 132.9669) centre (115.7787, 120.9669) ccw projected
  line L27 (127.7787, 120.9669) -> (-30.2213, 120.9669)
  line L28 (-30.2213, 120.9669) -> (-30.2213, 28.2)
  line L29 (-30.2213, 28.2) -> (-27.1, 28.2)
  line L30 (27.1, 24.9988) -> (27.1, -24.9988) projected
  line L31 (27.1, 0) -> (-27.1, 0)
  line L32 (127.7787, -120.9669) -> (-30.2213, -120.9669)
  line L33 (-30.2213, -120.9669) -> (-30.2213, -28.2)
  line L34 (-30.2213, -28.2) -> (-27.1, -28.2)
  arc A72 (-15.1, 132.9669) -> (-27.1, 120.9669) centre (-15.1, 120.9669) ccw projected
  line L35 (-15.1, 132.9669) -> (-30.2213, 132.9669)
  line L36 (-30.2213, 132.9669) -> (-30.2213, 120.9669)
  line L37 (-30.2213, -120.9669) -> (-30.2213, -132.9669)
  line L38 (115.7787, -132.9669) -> (-15.1, -132.9669) projected
  line L39 (-30.2213, -132.9669) -> (-15.1, -132.9669)
  line L40 (-27.1, 28.2) -> (27.5349, 28.2)
  arc A73 (34.6692, 36.1508) -> (27.1, 24.9988) centre (39.1, 24.9988) ccw projected
  line L41 (-27.1, -28.2) -> (27.5349, -28.2)
  arc A74 (27.1, -24.9988) -> (34.6692, -36.1508) centre (39.1, -24.9988) ccw projected
  line L42 (27.1, 24.9988) -> (27.1, -24.9988) projected
  line L43 (27.1, -24.9988) -> (27.1, -28.2)
  line L44 (27.1, 24.9988) -> (27.1, 28.2)
  line L45 (34.6692, 36.1508) -> (34.6692, -36.1508)
  point P0 (-27.1, -28.2)
  dimension "d323" = 28.2
  dimension "d324" = 28.2
  dimension "d325" = 158
  constraints: 36 end point, 7 point on line, 5 perpendicular, 3 horizontal, 2 midpoint, 2 point on circle, 2 symmetric about line, 1 parallel, 1 tangent
  measures "d323" distance of L24.start L24.end
  measures "d324" distance of L24.start L26.end
  measures "d325" distance of L13.end L27.end
extrude "돌출46" add sketch "스케치45" against normal blind 5 contours L32 L33 L34 L15 | A42 L39 L37 L32 | L29 L28 L27 L15 | A45 L11 A46 L45 | L27 L36 L35 A49
sketch "스케치47" plane through (0, 0, 0) normal (0, -1, 0) x (1, 0, 0)
  circle A0 centre (-18.1, 59.001) radius 1.6 projected
  circle A1 centre (17.9, 59.001) radius 1.6 projected
  circle A2 centre (114.8107, -128.501) radius 1.6 projected
  circle A3 centre (34.8107, -128.501) radius 1.6 projected
  circle A4 centre (49.8107, -128.501) radius 1.6 projected
  circle A5 centre (89.8107, -128.501) radius 1.6 projected
  circle A6 centre (4.8107, -128.501) radius 1.6 projected
  circle A7 centre (-15.1893, -128.501) radius 1.6 projected
  circle A8 centre (69.8107, -128.501) radius 1.6 projected
  circle A9 centre (-15.1893, -76.501) radius 1.6 projected
  circle A10 centre (69.8107, -76.501) radius 1.6 projected
  circle A11 centre (89.8107, -76.501) radius 1.6 projected
  circle A12 centre (4.8107, -76.501) radius 1.6 projected
  circle A13 centre (49.8107, -76.501) radius 1.6 projected
  circle A14 centre (114.8107, -76.501) radius 1.6 projected
  circle A15 centre (34.8107, -76.501) radius 1.6 projected
  circle A16 centre (34.8107, 76.501) radius 1.6 projected
  circle A17 centre (114.8107, 76.501) radius 1.6 projected
  circle A18 centre (49.8107, 76.501) radius 1.6 projected
  circle A19 centre (4.8107, 76.501) radius 1.6 projected
  circle A20 centre (89.8107, 76.501) radius 1.6 projected
  circle A21 centre (69.8107, 76.501) radius 1.6 projected
  circle A22 centre (-15.1893, 76.501) radius 1.6 projected
  circle A23 centre (-4.9749, 12.0104) radius 1.6 projected
  circle A24 centre (4.9749, 12.0104) radius 1.6 projected
  circle A25 centre (-12.0104, 4.9749) radius 1.6 projected
  circle A26 centre (12.0104, 4.9749) radius 1.6 projected
  line L0 (84.8787, -118.101) -> (50.8787, -118.101) projected
  arc A27 (47.8787, -115.101) -> (50.8787, -118.101) centre (50.8787, -115.101) ccw projected
  line L1 (47.8787, -115.101) -> (47.8787, -101.101) projected
  arc A28 (50.8787, -98.101) -> (47.8787, -101.101) centre (50.8787, -101.101) ccw projected
  line L2 (50.8787, -98.101) -> (84.8787, -98.101) projected
  arc A29 (87.8787, -101.101) -> (84.8787, -98.101) centre (84.8787, -101.101) ccw projected
  line L3 (87.8787, -101.101) -> (87.8787, -115.101) projected
  arc A30 (84.8787, -118.101) -> (87.8787, -115.101) centre (84.8787, -115.101) ccw projected
  circle A31 centre (69.8107, 128.501) radius 1.6 projected
  circle A32 centre (-15.1893, 128.501) radius 1.6 projected
  circle A33 centre (4.8107, 128.501) radius 1.6 projected
  circle A34 centre (89.8107, 128.501) radius 1.6 projected
  circle A35 centre (49.8107, 128.501) radius 1.6 projected
  circle A36 centre (34.8107, 128.501) radius 1.6 projected
  circle A37 centre (114.8107, 128.501) radius 1.6 projected
  line L4 (50.8787, 118.101) -> (84.8787, 118.101) projected
  arc A38 (87.8787, 115.101) -> (84.8787, 118.101) centre (84.8787, 115.101) ccw projected
  line L5 (87.8787, 115.101) -> (87.8787, 101.101) projected
  arc A39 (84.8787, 98.101) -> (87.8787, 101.101) centre (84.8787, 101.101) ccw projected
  line L6 (84.8787, 98.101) -> (50.8787, 98.101) projected
  arc A40 (47.8787, 101.101) -> (50.8787, 98.101) centre (50.8787, 101.101) ccw projected
  line L7 (47.8787, 101.101) -> (47.8787, 115.101) projected
  arc A41 (50.8787, 118.101) -> (47.8787, 115.101) centre (50.8787, 115.101) ccw projected
  line L8 (-30.2213, -132.9669) -> (115.7787, -132.9669) projected
  arc A42 (115.7787, -132.9669) -> (127.7787, -120.9669) centre (115.7787, -120.9669) ccw projected
  line L9 (127.7787, -120.9669) -> (127.7787, -81.2883) projected
  arc A43 (127.7787, -81.2883) -> (120.2094, -70.1362) centre (115.7787, -81.2883) ccw projected
  line L10 (120.2094, -70.1362) -> (34.6692, -36.1508) projected
  line L11 (34.6692, -36.1508) -> (34.6692, 36.1508) projected
  line L12 (34.6692, 36.1508) -> (120.2094, 70.1362) projected
  arc A44 (120.2094, 70.1362) -> (127.7787, 81.2883) centre (115.7787, 81.2883) ccw projected
  line L13 (127.7787, 81.2883) -> (127.7787, 120.9669) projected
  arc A45 (127.7787, 120.9669) -> (115.7787, 132.9669) centre (115.7787, 120.9669) ccw projected
  line L14 (115.7787, 132.9669) -> (-30.2213, 132.9669) projected
  line L15 (-30.2213, 132.9669) -> (-30.2213, 28.2) projected
  line L16 (-30.2213, 28.2) -> (-27.1, 28.2) projected
  line L17 (-27.1, 28.2) -> (-27.1, -28.2) projected
  line L18 (-27.1, -28.2) -> (-30.2213, -28.2) projected
  line L19 (-30.2213, -28.2) -> (-30.2213, -132.9669) projected
  circle A46 centre (99.9787, -108.101) radius 1.85 projected
  circle A47 centre (15.7787, 108.101) radius 1.85 projected
  circle A48 centre (35.7787, -108.101) radius 1.75 projected
  circle A49 centre (119.9787, 108.101) radius 1.75 projected
  circle A50 centre (119.9787, -108.101) radius 1.75 projected
  circle A51 centre (35.7787, 108.101) radius 1.75 projected
  circle A52 centre (15.7787, -108.101) radius 1.85 projected
  circle A53 centre (99.9787, 108.101) radius 1.85 projected
  circle A54 centre (0, 0) radius 8 projected
  arc A55 (13, 81.501) -> (15, 83.501) centre (13, 83.501) ccw projected
  line L20 (13, 81.501) -> (-13, 81.501) projected
  arc A56 (-15, 83.501) -> (-13, 81.501) centre (-13, 83.501) ccw projected
  line L21 (-15, 83.501) -> (-15, 93.501) projected
  arc A57 (-13, 95.501) -> (-15, 93.501) centre (-13, 93.501) ccw projected
  line L22 (-13, 95.501) -> (13, 95.501) projected
  arc A58 (15, 93.501) -> (13, 95.501) centre (13, 93.501) ccw projected
  line L23 (15, 93.501) -> (15, 83.501) projected
  circle A59 centre (-12.0104, -4.9749) radius 1.6 projected
  circle A60 centre (4.9749, -12.0104) radius 1.6 projected
  circle A61 centre (12.0104, -4.9749) radius 1.6 projected
  circle A62 centre (-4.9749, -12.0104) radius 1.6 projected
  line L24 (15, -83.501) -> (15, -93.501) projected
  arc A63 (13, -95.501) -> (15, -93.501) centre (13, -93.501) ccw projected
  line L25 (13, -95.501) -> (-13, -95.501) projected
  arc A64 (-15, -93.501) -> (-13, -95.501) centre (-13, -93.501) ccw projected
  line L26 (-15, -93.501) -> (-15, -83.501) projected
  arc A65 (-13, -81.501) -> (-15, -83.501) centre (-13, -83.501) ccw projected
  line L27 (-13, -81.501) -> (13, -81.501) projected
  arc A66 (15, -83.501) -> (13, -81.501) centre (13, -83.501) ccw projected
  line L28 (-27.1, -28.2) -> (-27.1, 28.2) projected
  line L29 (-27.1, 0) -> (-27.1, -54.2)
  line L30 (-27.1, 0) -> (27.1, 0)
  line L31 (27.1, 0) -> (27.1, -28.2)
  line L32 (27.1, -28.2) -> (34.6692, -28.2)
  line L33 (34.6692, 36.1508) -> (34.6692, -36.1508) projected
  line L34 (27.1, 0) -> (27.1, 28.2)
  line L35 (34.6692, 36.1508) -> (120.2094, 70.1362) projected
  line L36 (27.1, 28.2) -> (34.6692, 36.1508)
  line L37 (27.1, -28.2) -> (34.6692, -36.1508)
  line L38 (27.1, 28.2) -> (34.6692, 28.2)
  dimension "d331" = 54.2
  dimension "d332" = 54.2
  constraints: 16 end point, 3 point on line, 2 perpendicular, 1 collinear, 1 horizontal, 1 midpoint, 1 vertical
  measures "d331" distance of L29.start L29.end
  measures "d332" distance of L29.start L30.end
extrude "돌출47" cut sketch "스케치47" against normal blind 5 contours L32 L31 L34 L38 L11
fillet "모깎기9" radius 6 4 edges at (34.6692, 2.5, 36.1508) (34.6692, 2.5, -36.1508) (34.6692, 2.5, -28.2) (34.6692, 2.5, 28.2)
fillet "모깎기10" radius 12 2 edges at (-30.2213, 2.5, 132.9669) (-30.2213, 2.5, -132.9669)